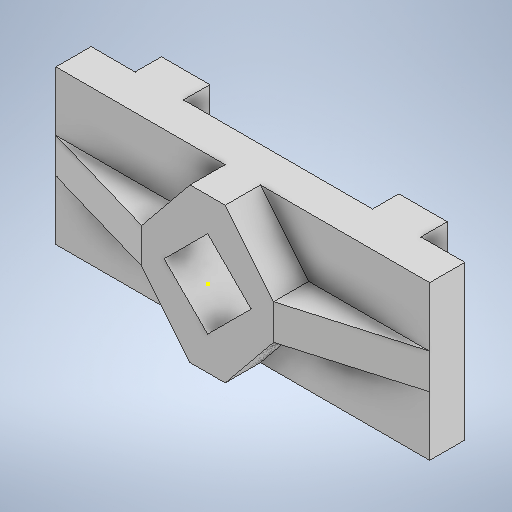
# Autodesk Inventor part: cad@44
Saved by Autodesk Inventor 2025.2 (Build 292293000, 293)
## iProperties
Created: 2025-04-01
Part Number: cad@44
Material: Generic
Document SubType Name: Modeling
Designer: spars
Density: 1 g/cm^3
Appearance: Default
Author: spars
Autodesk Inventor part; units mm, degrees
ref_plane "YZ Plane" through (0, 0, 0) normal (1, 0, 0) x (0, 1, 0)
ref_plane "XZ Plane" through (0, 0, 0) normal (0, 1, 0) x (-1, 0, 0)
ref_plane "XY Plane" through (0, 0, 0) normal (0, 0, 1) x (1, 0, 0)
sketch "Sketch1" plane through (0, 0, 0) normal (0, 0, 1) x (1, 0, 0)
  line L0 (-556.8071, 124.9561) -> (-221.4657, 119.2767) construction
  line L1 (-221.4657, 119.2767) -> (-225.781, -135.5254) construction
  line L2 (-225.781, -135.5254) -> (-561.1224, -129.8461) construction
  line L3 (-561.1224, -129.8461) -> (-556.8071, 124.9561) construction
  line L4 (-85, 35) -> (85, 35)
  line L5 (85, 35) -> (85, -35)
  line L6 (85, -35) -> (-85, -35)
  line L7 (-85, -35) -> (-85, 35)
  line L8 (-85, 35) -> (85, -35) construction
  line L9 (85, 35) -> (-85, -35) construction
  point P0 (0, 0)
  dimension "d13" = 170
  dimension "d14" = 70
  constraints: 12 end point, 2 midpoint, 2 parallel, 1 horizontal, 1 perpendicular, 2 other
  measures "d13" distance of L5.end L6.end
  measures "d14" distance of L4.end L5.end
extrude "Extrusion1" add sketch "Sketch1" along normal blind 16
sketch "Sketch2" plane through (0, 0, 0) normal (0, 0, -1) x (-1, 0, 0)
  line L0 (-85, 35) -> (85, 35) projected
  line L1 (-69.3459, 35) -> (0.6541, 35)
  line L2 (85, -35) -> (-85, -35) projected
  line L3 (-65, 35) -> (-43, 35)
  line L4 (-43, 35) -> (-43, -35)
  line L5 (-43, -35) -> (-65, -35)
  line L6 (-65, -35) -> (-65, 35)
  line L7 (-85, -35) -> (-85, 35) projected
  line L8 (85, 35) -> (-85, 35)
  line L9 (-85, -35) -> (85, -35)
  line L10 (43, 35) -> (43, -35)
  line L11 (65, -35) -> (65, 35)
  point P0 (0, 0)
  dimension "d17" = 70
  dimension "d18" = 22
  dimension "d19" = 20
  constraints: 18 end point, 5 point on line, 2 parallel, 1 horizontal, 1 perpendicular
  measures "d17" distance of L1.start L1.end
  measures "d18" distance of L4.end L5.end
  measures "d19" distance between parallel lines of L7 L6
extrude "Extrusion2" add sketch "Sketch2" along normal blind 12 contours L0 L4 L2 L6 | L10 L0 L11 L2
sketch "Sketch3" plane through (0, 0, 16) normal (0, 0, 1) x (1, 0, 0)
  line L0 (-8, 35) -> (8, 35)
  line L1 (30, 8) -> (30, -8)
  line L2 (8, -35) -> (-8, -35)
  line L3 (-30, -8) -> (-30, 8)
  line L4 (-30, 35) -> (30, -35) construction
  line L5 (30, 35) -> (-30, -35) construction
  line L6 (-8, 35) -> (-30, 8)
  line L7 (-8, -35) -> (-30, -8)
  line L8 (8, -35) -> (30, -8)
  line L9 (8, 35) -> (30, 8)
  point P0 (0, 0)
  dimension "d22" = 60
  dimension "d23" = 70
  dimension "d24" = 22
  dimension "d25" = 27
  dimension "d26" = 22
  dimension "d27" = 27
  dimension "d28" = 22
  dimension "d29" = 27
  dimension "d30" = 22
  dimension "d31" = 27
  constraints: 20 end point, 8 point on line, 2 midpoint, 2 parallel, 1 horizontal, 1 perpendicular
  measures "d22" distance of L4.end L5.end
  measures "d23" distance of L5.start L4.end
  measures "d24" distance of L0.start L4.start
  measures "d25" distance of L3.end L4.start
  measures "d26" distance of L2.end L5.end
  measures "d27" distance of L3.start L5.end
  measures "d28" distance of L2.start L4.end
  measures "d29" distance of L1.end L4.end
  measures "d30" distance of L0.end L5.start
  measures "d31" distance of L1.start L5.start
extrude "Extrusion3" add sketch "Sketch3" along normal blind 16
sketch "Sketch4" plane through (0, 0, 0) normal (0, 1, 0) x (-1, 0, 0)
  line L0 (85, 0) -> (85, 16) projected
  line L1 (8, 32) -> (30, 32) projected
  line L2 (70.4877, 20.2217) -> (52.5654, 25.4355)
  point P0 (0, 0)
  constraints: 2 end point
extrude "Rib1" add sketch "Sketch4" along normal mid plane 16 rib yes fills toward (61.5126, 22.7806) open curves L2
sketch "Sketch5" plane through (0, 0, 0) normal (0, 1, 0) x (-1, 0, 0)
  line L0 (-30, 32) -> (-8, 32) projected
  line L1 (-85, 0) -> (-85, 16) projected
  line L2 (-45.638, 27.4508) -> (-64.4396, 21.9812)
  point P0 (0, 0)
  constraints: 2 end point
extrude "Rib2" add sketch "Sketch5" along normal mid plane 16 rib yes fills toward (-55.0249, 24.668) open curves L2
sketch "Sketch6" plane through (0, 0, 32) normal (0, 0, 1) x (1, 0, 0)
  line L0 (-19.799, 0) -> (0, 19.799)
  line L1 (0, 19.799) -> (19.799, 0)
  line L2 (19.799, 0) -> (0, -19.799)
  line L3 (0, -19.799) -> (-19.799, 0)
  line L4 (-14, 14) -> (14, -14) construction
  line L5 (14, 14) -> (-14, -14) construction
  point P0 (0, 0)
  dimension "d46" = 28
  dimension "d47" = 28
  constraints: 12 end point, 2 midpoint, 2 parallel, 1 perpendicular
  measures "d46" distance of L1.end L2.end
  measures "d47" distance of L0.end L1.end
extrude "Extrusion4" cut sketch "Sketch6" against normal through all
sketch "Sketch7" plane through (0, 0, 32) normal (0, 0, 1) x (1, 0, 0)
  point P0 (0, 0)
equation "\"d26\" = d24"
equation "\"d27\" = d25"
equation "\"d28\" = d24"
equation "\"d29\" = d25"
equation "\"d30\" = d24"
equation "\"d31\" = d25"
body "Solid1"
